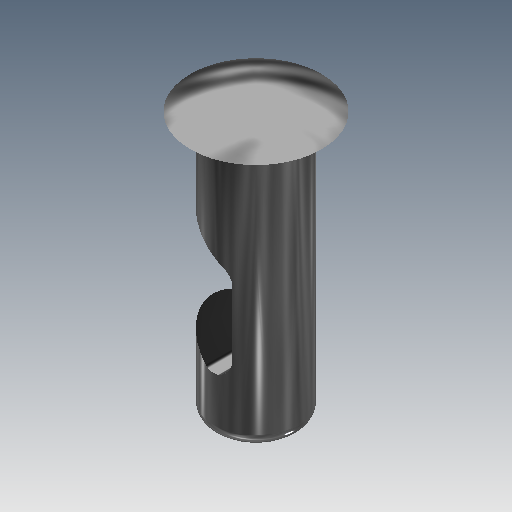
# Autodesk Inventor part: Pin
Saved by Autodesk Inventor 2020.1 (Build 241239000, 239)
## iProperties
Created: 2010-10-13
Part Number: Pin
Document SubType Name: Modeling
Designer: Thom Tremblay
Density: 1 g/cm^3
Material: Generic
Appearance: Chrome - Polished Black
Author: Thom Tremblay
Autodesk Inventor part; units mm, degrees
ref_plane "YZ Plane" through (0, 0, 0) normal (1, 0, 0) x (0, 1, 0)
ref_plane "XZ Plane" through (0, 0, 0) normal (0, 1, 0) x (-1, 0, 0)
ref_plane "XY Plane" through (0, 0, 0) normal (0, 0, 1) x (1, 0, 0)
sketch "Sketch1" plane through (0, 0, 0) normal (0, 0, 1) x (1, 0, 0)
  line L0 (0, 0) -> (0, 0.254)
  arc A0 (0, 0.254) -> (-1.27, -0.027) centre (0, -2.7564) ccw
  line L1 (-1.27, -0.027) -> (-0.8255, -0.027)
  line L2 (-0.8255, -0.027) -> (-0.8255, -5.0969)
  line L3 (0, -5.08) -> (0, 0)
  line L4 (0, -5.08) -> (0, -5.1562)
  arc A1 (-0.8255, -5.0969) -> (0, -5.1562) centre (0, 0.6234) ccw
  dimension "d0" = 1.651
  dimension "d1" = 2.54
  dimension "d2" = 5.08
  dimension "d3" = 0.254
  dimension "d4" = 0.0762
  constraints: 10 end point, 4 point on circle, 2 centre point, 2 collinear, 2 point on line, 1 parallel, 1 perpendicular, 1 vertical
  measures "d0" diameter of L2 L3
  measures "d1" diameter of L1.start L3
  measures "d2" distance of L3.start L0.start
  measures "d3" distance of L0.start L0.end
  measures "d4" distance of L3.start L4.end
revolve "Revolution1" add sketch "Sketch1" angle 360 about axis through (0, -5.08, 0) along (0, 1, 0)
sketch "Sketch2" plane through (0, 0, 0) normal (0, 0, 1) x (1, 0, 0)
  line L0 (-0.8255, -5.0969) -> (-0.8255, -0.027) projected
  line L1 (0, -4.572) -> (0, 0.762) construction
  line L2 (-0.8255, -3.494) -> (-0.1748, -3.9496)
  arc A0 (-0.1748, -3.9496) -> (0.3048, -3.6999) centre (0, -3.6999) ccw
  line L3 (0.3048, -3.6999) -> (0.3048, -2.4121)
  arc A1 (0.3048, -2.4121) -> (0.1748, -2.1624) centre (0, -2.4121) ccw
  line L4 (0.1748, -2.1624) -> (-0.8255, -1.462)
  point P0 (0, 0)
  dimension "d6" = 0.3048
  dimension "d7" = 55
  dimension "d8" = 55
  dimension "d11" = 1.397
  dimension "d12" = 2.032
  constraints: 6 end point, 4 point on circle, 4 point on line, 4 tangent, 2 centre point, 2 parallel
  measures "d6" radius of A0
  measures "d7" angle of L1 L2
  measures "d8" angle of L1 L4
  measures "d11" vertical distance of L0.start A0.centre
  measures "d12" distance of L2.start L4.end
extrude "Extrusion1" cut sketch "Sketch2" along normal through all both and the other way through all
fillet "Fillet1" radius 0.254 1 edges at (0.8255, -5.0969, 0)
body "Solid1"
